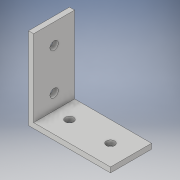
# Autodesk Inventor part: LV Gusset
Saved by Autodesk Inventor 2018 (Build 220112000, 112)
## iProperties
Created: 2019-01-25
Part Number: LV Gusset
Material: Generic
Document SubType Name: Modeling
Designer: Gabriel
Density: 1 g/cm^3
Appearance: Default
Author: Gabriel
Autodesk Inventor part; units mm, degrees
ref_plane "YZ Plane" through (0, 0, 0) normal (1, 0, 0) x (0, 1, 0)
ref_plane "XZ Plane" through (0, 0, 0) normal (0, 1, 0) x (-1, 0, 0)
ref_plane "XY Plane" through (0, 0, 0) normal (0, 0, 1) x (1, 0, 0)
sketch "Sketch1" plane through (0, 0, 0) normal (0, 0, 1) x (1, 0, 0)
  line L0 (0, 0) -> (3.175, 0)
  line L1 (3.175, 0) -> (3.175, 50.8)
  line L2 (3.175, 50.8) -> (0, 50.8)
  line L3 (0, 50.8) -> (0, 0)
  line L4 (0, 0) -> (50.8, 0)
  line L5 (50.8, 0) -> (50.8, 3.175)
  line L6 (50.8, 3.175) -> (0, 3.175)
  line L7 (0, 3.175) -> (0, 0)
  dimension "d0" = 3.175
  dimension "d1" = 50.8
  dimension "d2" = 50.8
  dimension "d3" = 3.175
  constraints: 16 end point, 4 parallel, 2 horizontal, 2 perpendicular
  measures "d0" distance of L2.end L1.end
  measures "d1" distance of L1.end L0.end
  measures "d2" distance of L6.end L5.end
  measures "d3" distance of L5.end L4.end
extrude "Extrusion1" add sketch "Sketch1" along normal blind 25.4
sketch "Sketch2" plane through (3.175, 3.175, 0) normal (1, 0, 0) x (0, 0, -1)
  line L0 (0, 47.625) -> (-25.4, 47.625) construction
  line L1 (0, 0) -> (-25.4, 0) construction
  line L2 (-12.7, 0) -> (-12.7, 9.525) construction
  circle A0 centre (-12.7, 9.525) radius 2.5797
  line L3 (-12.7, 9.525) -> (-12.7, 34.925) construction
  circle A1 centre (-12.7, 34.925) radius 2.5797
  point P0 (0, -3.175)
  dimension "d18" = 9.525
  dimension "d19" = 5.1594
  dimension "d22" = 25.4
  dimension "d23" = 5.1594
  constraints: 4 end point, 2 centre point, 2 coincident, 2 vertical, 1 midpoint
  measures "d18" distance of L2.start L2.end
  measures "d19" diameter of A0
  measures "d22" distance of L3.start L3.end
  measures "d23" diameter of A1
extrude "Extrusion2" cut sketch "Sketch2" against normal blind 25.4
sketch "Sketch3" plane through (3.175, 3.175, 0) normal (0, 1, 0) x (1, 0, 0)
  line L0 (0, 0) -> (0, -25.4) construction
  line L1 (0, -12.7) -> (9.525, -12.7) construction
  circle A0 centre (9.525, -12.7) radius 2.5797
  line L2 (9.525, -12.7) -> (34.925, -12.7) construction
  circle A1 centre (34.925, -12.7) radius 2.5797
  point P0 (-3.175, 0)
  dimension "d12" = 9.525
  dimension "d13" = 5.1594
  dimension "d14" = 25.4
  dimension "d15" = 5.1594
  constraints: 4 end point, 2 centre point, 2 coincident, 2 horizontal, 1 midpoint
  measures "d12" distance of L1.start L1.end
  measures "d13" diameter of A0
  measures "d14" distance of L2.start L2.end
  measures "d15" diameter of A1
extrude "Extrusion3" cut sketch "Sketch3" against normal blind 25.4
body "Solid1"
